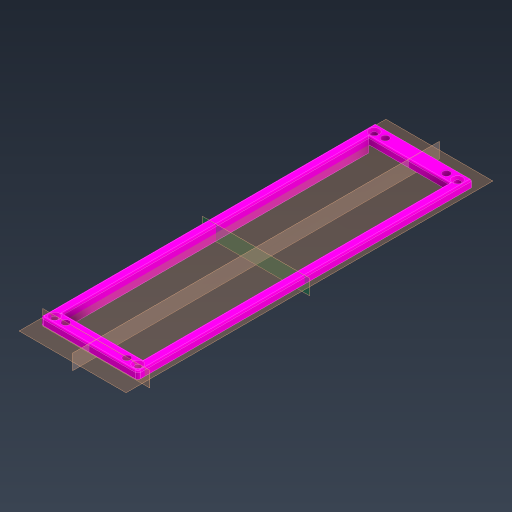
# Autodesk Inventor part: Проставка_крепления_ динамика
Saved by Autodesk Inventor 2023.2 (Build 272271030, 271C)
## iProperties
Created: 2025-09-19
Part Number: Проставка_крепления_ динамика
Material: Типовые
Document SubType Name: Modeling
Designer: Олег Коноваленко
Density: 1 g/cm^3
Appearance: Пурпурный
Author: Олег Коноваленко
Autodesk Inventor part; units mm, degrees
sketch "Эскиз1" plane through (0, 0, 0) normal (0, 1, 0) x (-1, 0, 0)
  line L0 (35, 5) -> (-35, 5)
  line L1 (-35, 5) -> (-35, -5)
  line L2 (-35, -5) -> (35, -5)
  line L3 (35, -5) -> (35, 5)
  line L4 (35, 5) -> (-35, -5) construction
  line L5 (-35, 5) -> (35, -5) construction
  point P0 (0, 0)
  dimension "d0" = 70
  dimension "d1" = 10
  constraints: 12 end point, 2 midpoint, 2 parallel, 1 horizontal, 1 perpendicular
  measures "d0" distance of L1.end L2.end
  measures "d1" distance of L0.end L1.end
extrude "Выдавливание1" add sketch "Эскиз1" along normal blind 5
sketch "Эскиз2" plane through (0, 5, 0) normal (0, 1, 0) x (1, 0, 0)
  circle A0 centre (30, 0) radius 2.55 projected
  circle A1 centre (-30, 0) radius 2.55 projected
  circle A2 centre (30, 0) radius 2.1
  circle A3 centre (-30, 0) radius 2.1
  point P0 (0, 0)
  dimension "d4" = 4.2
  constraints: 2 centre point, 2 coincident, 1 equal radius
  measures "d4" diameter of A2
fillet "Сопряжение1" radius 2 2 edges at (-35, 2.5, 5) (35, 2.5, 5)
extrude "Выдавливание2" cut sketch "Эскиз2" against normal up to next contours A2 | A3
sketch "Эскиз3" plane through (0, 5, 0) normal (0, 1, 0) x (1, 0, 0)
  line L0 (35, 5) -> (-35, 5) projected
  line L1 (35, 5) -> (35, 115)
  line L2 (49, 115) -> (-49, 115)
  line L3 (-35, 5) -> (-35, -3) projected
  line L4 (-35, 5) -> (-35, 115)
  line L5 (-28.6816, 115) -> (-28.6816, 5) projected
  line L6 (28.6816, 115) -> (28.6816, 5) projected
  point P0 (0, 0)
  constraints: 6 end point, 2 point on line, 1 horizontal, 1 perpendicular, 1 vertical, 2 other
extrude "Выдавливание3" add sketch "Эскиз3" against normal blind 5 contours L0 L6 L2 L1 | L0 L4 L2 L5
sketch "Эскиз4" plane through (0, 0, 0) normal (0, -1, 0) x (1, 0, 0)
  line L0 (28.6816, -115) -> (31.1816, -115)
  line L1 (31.1816, -115) -> (31.1816, -5)
  line L2 (31.1816, -5) -> (28.6816, -5)
  line L3 (28.6816, -5) -> (28.6816, -115)
  line L4 (0, 29) -> (0, -139) projected
  line L5 (-28.6816, -115) -> (-31.1816, -115)
  line L6 (-31.1816, -115) -> (-31.1816, -5)
  line L7 (-31.1816, -5) -> (-28.6816, -5)
  line L8 (-28.6816, -5) -> (-28.6816, -115)
  point P0 (0, 0)
  dimension "d10" = 2.5
  constraints: 16 end point, 5 symmetric about line, 2 parallel, 2 point on line, 1 horizontal, 1 perpendicular
  measures "d10" distance of L0.start L0.end
extrude "Выдавливание4" add sketch "Эскиз4" along normal blind 5
chamfer "Фаска1" distance 1.5 angle 45 2 edges at (27.9, 5, 0) (-32.1, 5, 0)
sketch "Эскиз5" plane through (0, 5, 0) normal (0, 1, 0) x (1, 0, 0)
  circle A0 centre (22, 0) radius 2.55
  circle A1 centre (-22, 0) radius 2.55
  circle A2 centre (30, 0) radius 2.1 projected
  circle A3 centre (-30, 0) radius 2.1 projected
  point P0 (0, 0)
  dimension "d16" = 8
  dimension "d17" = 8
  dimension "d18" = 5.1
  constraints: 2 centre point, 1 equal radius
  measures "d16" distance of A2.centre A0.centre
  measures "d17" distance of A3.centre A1.centre
  measures "d18" diameter of A0
extrude "Выдавливание5" cut sketch "Эскиз5" against normal up to next contours A0 | A1
ref_plane "РабПлоскость1" through (-31.1816, 0, -115) normal (0, 0, -1) x (-1, 0, 0)
mirror "Зеркальное отражение1" about plane through (-31.1816, 0, -115) normal (0, 0, -1) of "Выдавливание1", "Фаска1", "Выдавливание5", "Выдавливание2", "Выдавливание3", "Выдавливание4"
fillet "Сопряжение2" radius 2 6 edges at (-31.1816, -2.5, -5) (-31.1816, -2.5, -225) (31.1816, -2.5, -225) (31.1816, -2.5, -5) (-31.1816, -5, -115) (31.1816, -5, -115)
fillet "Сопряжение3" radius 1 9 edges at (34.4142, 5, 4.4142) (0, 5, 5) (-34.4142, 5, 4.4142) (-35, 5, -116) (35, 5, -116) (-28.6816, 5, -115) (0, 5, -5) (28.6816, 5, -115) (0, 5, -225)
chamfer "Фаска2" distance 0.5 angle 45 5 edges at (-31.1816, 0, -115) (-30.5959, 0, -5.5858) (-28.9316, 0, -5) (-30.5959, 0, -224.4142) (-28.9316, 0, -225)
chamfer "Фаска3" distance 0.5 angle 45 5 edges at (31.1816, 0, -115) (30.5959, 0, -5.5858) (28.9316, 0, -5) (30.5959, 0, -224.4142) (28.9316, 0, -225)
